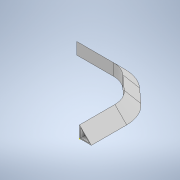
# Autodesk Inventor part: lab_4_4
Saved by Autodesk Inventor 2020 (Build 240168000, 168)
## iProperties
Created: 2020-03-31
Part Number: lab_4_4
Material: Типовые
Document SubType Name: Modeling
Designer: User
Density: 1 g/cm^3
Appearance: По умолчанию
Author: User
Autodesk Inventor part; units mm, degrees
ref_plane "YZ Plane" through (0, 0, 0) normal (1, 0, 0) x (0, 1, 0)
ref_plane "XZ Plane" through (0, 0, 0) normal (0, 1, 0) x (-1, 0, 0)
ref_plane "XY Plane" through (0, 0, 0) normal (0, 0, 1) x (1, 0, 0)
sketch "Эскиз1" plane through (0, 0, 0) normal (0, 0, 1) x (1, 0, 0)
  line L0 (0, 0) -> (0, 130)
  line L1 (0, 0) -> (130, 0)
  line L2 (130, 0) -> (0, 130)
  dimension "d0" = 130
  dimension "d1" = 130
  constraints: 6 end point, 1 horizontal, 1 vertical
  measures "d0" distance of L0.start L0.end
  measures "d1" distance of L0.start L1.end
sketch "Эскиз2" plane through (0, 0, 0) normal (0, 1, 0) x (-1, 0, 0)
  point P0 (0, 0)
sketch "Эскиз3" plane through (0, 0, 0) normal (0, 1, 0) x (-1, 0, 0)
  point P0 (0, 0)
sketch "Эскиз4" plane through (0, 0, 0) normal (0, 0, 1) x (1, 0, 0)
  line L0 (0, 0) -> (10, 0)
  line L1 (10, 10) -> (10, 110)
  line L2 (10, 10) -> (110, 10)
  line L3 (110, 10) -> (10, 110)
  dimension "d3" = 10
  dimension "d4" = 100
  dimension "d5" = 100
  constraints: 8 end point, 2 horizontal
  measures "d3" distance of L0.end L1.start
  measures "d4" distance of L1.start L1.end
  measures "d5" distance of L1.start L2.end
sketch "Эскиз5" plane through (0, 0, 0) normal (0, 1, 0) x (-1, 0, 0)
  line L0 (0, 0) -> (0, -388.8774)
  line L1 (82.4884, -574.4573) -> (238.5702, -715.3428)
  line L2 (406.0818, -779.7629) -> (809.939, -779.7629)
  arc A0 (0, -388.8774) -> (82.4884, -574.4573) centre (250, -388.8774) ccw
  arc A1 (238.5702, -715.3428) -> (406.0818, -779.7629) centre (406.0818, -529.7629) ccw
  point P0 (0, -500)
  point P1 (309.939, -779.7629)
  dimension "d6" = 500
  dimension "d7" = 500
  dimension "d8" = 250
  constraints: 6 end point, 4 point on circle, 4 point on line, 4 tangent, 2 centre point, 1 equal radius, 1 perpendicular, 1 vertical
  measures "d6" distance of L0.start point (0, -500)
  measures "d7" distance of point (309.939, -779.763) L2.end
  measures "d8" radius of A0
sketch "Эскиз6" plane through (0, 0, 0) normal (0, 1, 0) x (-1, 0, 0)
  point P0 (0, 0)
sketch "Эскиз7" plane through (0, 0, 0) normal (0, 0, 1) x (1, 0, 0)
  point P0 (0, 0)
sweep "Сдвиг1" add profiles "Эскиз1" path "Эскиз5"
sketch3d "3D эскиз1"
  line L0 (0, 0, 0) -> (0, 0, -388.8774)
  arc A0 (0, 0, -388.8774) -> (-82.4884, 0, -574.4573) centre (-250, 0, -388.8774) ccw
  line L1 (-82.4884, 0, -574.4573) -> (-238.5702, 0, -715.3428)
  arc A1 (-238.5702, 0, -715.3428) -> (-406.0818, 0, -779.7629) centre (-406.0818, 0, -529.7629) ccw
  line L2 (-406.0818, 0, -779.7629) -> (-809.939, 0, -779.7629)
sweep "Сдвиг2" cut profiles "Эскиз4" path "3D эскиз1"
